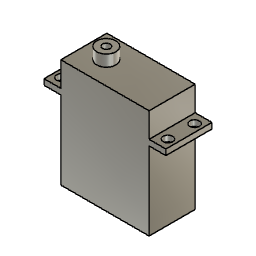
SCS2332舵机 v2 (Autodesk Fusion 360 design; units mm, degrees)
Autodesk Fusion 360 part; units mm, degrees
sketch "草图1" plane through (0, 0, 0) normal (0, 0, 1) x (1, 0, 0)
  line L0 (16, -6.05) -> (-16, -6.05)
  line L1 (-16, -6.05) -> (-16, 6.05)
  line L2 (-16, 6.05) -> (16, 6.05)
  line L3 (16, 6.05) -> (16, -6.05)
  line L4 (16, -6.05) -> (-16, 6.05) construction
  line L5 (-16, -6.05) -> (16, 6.05) construction
  line L6 (-18, 0) -> (25, 0)
  line L7 (0, 20) -> (0, -24)
  circle A0 centre (-14, 3.5) radius 1.25
  circle A1 centre (14, 3.5) radius 1.25
  circle A2 centre (-14, -3.5) radius 1.25
  circle A3 centre (14, -3.5) radius 1.25
  dimension "d1" = 12.1
  dimension "d2" = 32
  dimension "d4" = 2.5
  dimension "d5" = 28
  dimension "d6" = 7
  constraint horizontal L0
  constraint perpendicular L0 L1
  constraint parallel L0 L2
  constraint parallel L1 L3
  constraint coincident L4 origin
  constraint coincident L5 origin
  constraint perpendicular L1 L6
  constraint perpendicular L2 L7
  constraint symmetric L1 L3 L7
  constraint symmetric L0 L2 L6
  constraint symmetric L7 A0 A1
  constraint symmetric L6 A0 A2
  constraint symmetric L6 A1 A3
  measures "d1" distance of L0.end L1.end
  measures "d2" distance of L1.end L2.end
  measures "d4" diameter of A0
  measures "d5" distance of A0.centre A1.centre
  measures "d6" distance of A0.centre A2.centre
extrude "拉伸1" add sketch "草图1" along normal blind 1.5 makes body 1
sketch "草图2" plane through (0, 0, 0) normal (0, 0, -1) x (1, 0, 0)
  circle A0 centre (14, -3.5) radius 1.25
  circle A1 centre (-14, -3.5) radius 1.25
  circle A2 centre (-14, 3.5) radius 1.25
  circle A3 centre (14, 3.5) radius 1.25
  line L0 (-16, -6.05) -> (16, -6.05)
  line L1 (16, -6.05) -> (16, 6.05)
  line L2 (16, 6.05) -> (-16, 6.05)
  line L3 (-16, 6.05) -> (-16, -6.05)
  line L4 (11.6, -6.05) -> (-11.6, -6.05)
  line L5 (-11.6, -6.05) -> (-11.6, 6.05)
  line L6 (-11.6, 6.05) -> (11.6, 6.05)
  line L7 (11.6, 6.05) -> (11.6, -6.05)
  line L8 (11.6, -6.05) -> (-11.6, 6.05) construction
  line L9 (-11.6, -6.05) -> (11.6, 6.05) construction
  dimension "d9" = 23.2
  dimension "d10" = 12.1
  constraint horizontal L4
  constraint perpendicular L4 L5
  constraint parallel L4 L6
  constraint parallel L5 L7
  constraint coincident L8 origin
  constraint coincident L9 origin
  measures "d9" distance of L5.end L6.end
  measures "d10" distance of L4.start L6.end
extrude "拉伸2" add sketch "草图2" along normal blind 20.5 contours L0 L2 L4 L5 L6 L7 bodies 1
sketch "草图3" plane through (0, 0, 1.5) normal (0, 0, 1) x (-1, 0, 0)
  circle A0 centre (14, 3.5) radius 1.25
  circle A1 centre (-14, 3.5) radius 1.25
  circle A2 centre (-14, -3.5) radius 1.25
  circle A3 centre (14, -3.5) radius 1.25
  line L0 (-16, -6.05) -> (16, -6.05)
  line L1 (16, -6.05) -> (16, 6.05)
  line L2 (16, 6.05) -> (-16, 6.05)
  line L3 (-16, 6.05) -> (-16, -6.05)
  line L4 (-11.6, 6.05) -> (11.6, 6.05)
  line L5 (11.6, 6.05) -> (11.6, -6.05)
  line L6 (11.6, -6.05) -> (-11.6, -6.05)
  line L7 (-11.6, -6.05) -> (-11.6, 6.05)
  line L8 (-11.6, 6.05) -> (11.6, -6.05) construction
  line L9 (11.6, 6.05) -> (-11.6, -6.05) construction
  dimension "d13" = 23.2
  dimension "d14" = 12.1
  constraint horizontal L4
  constraint perpendicular L4 L5
  constraint parallel L4 L6
  constraint parallel L5 L7
  constraint coincident L8 origin
  constraint coincident L9 origin
  constraint coincident L2 L4.start
  measures "d13" distance of L5.end L6.end
  measures "d14" distance of L4.start L6.end
extrude "拉伸3" add sketch "草图3" along normal blind 6.5 contours L0 L2 L4 L5 L6 L7 bodies 1
sketch "草图4" plane through (0, 0, 8) normal (0, 0, 1) x (-1, 0, 0)
  line L0 (-11.6, -6.05) -> (11.6, -6.05)
  line L1 (11.6, -6.05) -> (11.6, 6.05)
  line L2 (11.6, 6.05) -> (-11.6, 6.05)
  line L3 (-11.6, 6.05) -> (-11.6, -6.05)
  line L4 (11.6, 6.05) -> (11.6, -6.05)
  line L5 (11.6, -6.05) -> (16, -6.05)
  line L6 (16, -6.05) -> (16, 6.05)
  line L7 (16, 6.05) -> (11.6, 6.05)
  circle A0 centre (14, -3.5) radius 1.25
  circle A1 centre (14, 3.5) radius 1.25
  line L8 (-11.6, -6.05) -> (-11.6, 6.05)
  line L9 (-11.6, 6.05) -> (-16, 6.05)
  line L10 (-16, 6.05) -> (-16, -6.05)
  line L11 (-16, -6.05) -> (-11.6, -6.05)
  circle A2 centre (-14, 3.5) radius 1.25
  circle A3 centre (-14, -3.5) radius 1.25
  circle A4 centre (5.7, 0) radius 2.5
  circle A5 centre (5.7, 0) radius 1
  dimension "d17" = 5
  dimension "d18" = 8.3
  dimension "d19" = 2
  constraint concentric A4 A5
  measures "d17" diameter of A4
  measures "d18" horizontal distance of A0.centre A4.centre
  measures "d19" diameter of A5
extrude "拉伸4" add sketch "草图4" along normal blind 3 separate body contours A4 makes body 2
